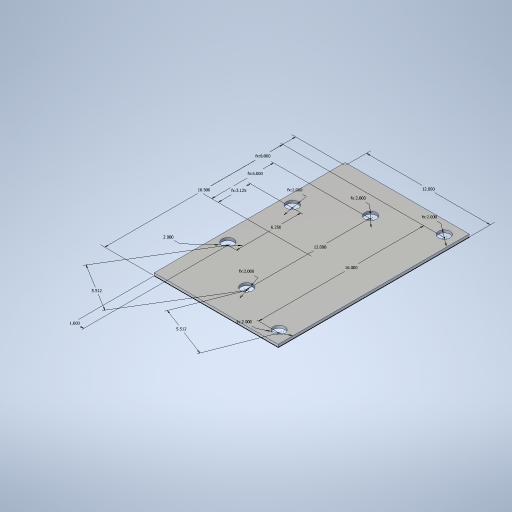
# Autodesk Inventor part: Int1-001
Saved by Autodesk Inventor 2023.4 (Build 274418000, 418)
## iProperties
Created: 2025-01-15
Part Number: Int1-001
Material: Aluminum 6061
Document SubType Name: Modeling
Designer: mavericks
Density: 2.7 g/cm^3
Appearance: Aluminum - Flat
Author: mavericks
Autodesk Inventor part; units mm, degrees
ref_plane "YZ Plane" through (0, 0, 0) normal (1, 0, 0) x (0, 1, 0)
ref_plane "XZ Plane" through (0, 0, 0) normal (0, 1, 0) x (-1, 0, 0)
ref_plane "XY Plane" through (0, 0, 0) normal (0, 0, 1) x (1, 0, 0)
sketch "Sketch1" plane through (0, 0, 0) normal (0, 1, 0) x (-1, 0, 0)
  line L0 (-152.4, 234.95) -> (152.4, 234.95)
  line L1 (152.4, 234.95) -> (152.4, -234.95)
  line L2 (152.4, -234.95) -> (-152.4, -234.95)
  line L3 (-152.4, -234.95) -> (-152.4, 234.95)
  line L4 (-152.4, 234.95) -> (152.4, -234.95) construction
  line L5 (152.4, 234.95) -> (-152.4, -234.95) construction
  circle A0 centre (127, -79.375) radius 25.4 construction
  circle A1 centre (127, 79.375) radius 25.4 construction
  circle A2 centre (7.5484, 152.4) radius 25.4 construction
  circle A3 centre (7.5484, -152.4) radius 25.4 construction
  circle A4 centre (-122.9151, -203.2) radius 25.4 construction
  circle A5 centre (-122.9151, 203.2) radius 25.4 construction
  point P0 (0, 0)
  dimension "d0" = 304.8
  dimension "d1" = 469.9
  dimension "d2" = 158.75
  dimension "d3" = 50.8
  dimension "d4" = 50.8
  dimension "d5" = 79.375
  dimension "d6" = 50.8
  dimension "d7" = 50.8
  dimension "d8" = 50.8
  dimension "d9" = 50.8
  dimension "d10" = 406.4
  dimension "d11" = 304.8
  dimension "d12" = 152.4
  dimension "d14" = 203.2
  dimension "d17" = 140.0048
  dimension "d18" = 140.0048
  dimension "d19" = 25.4
  constraints: 12 end point, 6 centre point, 6 coincident, 3 vertical alignment, 2 midpoint, 2 parallel, 1 horizontal, 1 perpendicular
  measures "d0" distance of L1.end L2.end
  measures "d1" distance of L0.end L1.end
  measures "d2" distance of point (127, -79.375) point (127, 79.375)
  measures "d3" diameter of A0
  measures "d4" diameter of A1
  measures "d5" vertical distance of point (127, -79.375) point (0, 0)
  measures "d6" diameter of A2
  measures "d7" diameter of A3
  measures "d8" diameter of A4
  measures "d9" diameter of A5
  measures "d10" distance of point (-122.915, -203.2) point (-122.915, 203.2)
  measures "d11" distance of point (7.548, -152.4) point (7.548, 152.4)
  measures "d12" vertical distance of point (7.548, -152.4) point (0, 0)
  measures "d14" vertical distance of point (-122.915, -203.2) point (0, 0)
  measures "d17" distance of point (7.548, 152.4) point (127, 79.375)
  measures "d18" distance of point (-122.915, 203.2) point (7.548, 152.4)
  measures "d19" distance from line of L1 point (127, 79.375)
extrude "Extrusion1" add sketch "Sketch1" along normal blind 6.35
hole "Hole1" at (-127, 0, 79.375) at (-127, 0, -79.375) at (-7.5484, 0, 152.4) at (122.9151, 0, 203.2) at (-7.5484, 0, -152.4) at (122.9151, 0, -203.2) direction (0, 1, 0) diameter 28.575 end through all
equation "\"d3\" = d4"
equation "\"d5\" = 0.5 * d2"
equation "\"d6\" = d4"
equation "\"d7\" = d4"
equation "\"d8\" = d4"
equation "\"d9\" = d4"
equation "\"d12\" = 0.5 * d11"
equation "\"d14\" = 0.5 * d10"
body "Solid1"
